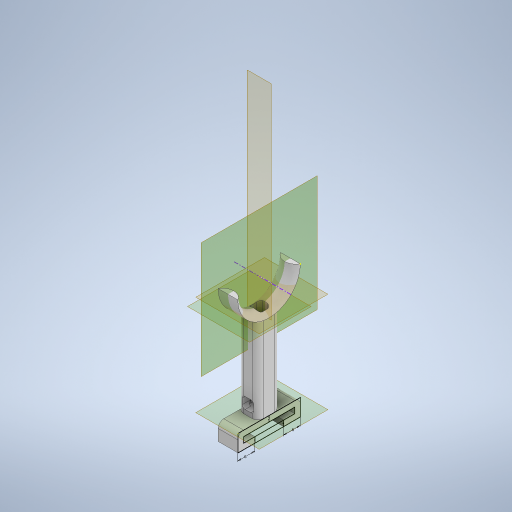
# Autodesk Inventor part: 막대1
Saved by Autodesk Inventor 2023 (Build 270158000, 158)
## iProperties
Created: 2023-04-26
Part Number: 막대1
Material: 일반
Document SubType Name: Modeling
Designer: rlatk
Density: 1 g/cm^3
Appearance: 기본값
Author: rlatk
Autodesk Inventor part; units mm, degrees
ref_plane "YZ Plane" through (0, 0, 0) normal (1, 0, 0) x (0, 1, 0)
ref_plane "XZ Plane" through (0, 0, 0) normal (0, 1, 0) x (-1, 0, 0)
sketch "스케치1" plane through (0, 0, 0) normal (0, 1, 0) x (-1, 0, 0)
  line L0 (0, 0) -> (3.5, 0)
  line L1 (0, 0) -> (-3.5, 0)
  arc A0 (3.5, 0) -> (-3.5, 0) centre (0, -1.9365) ccw
  line L2 (3.5, 0) -> (-3.5, 0)
  dimension "d1" = 3.5
  dimension "d2" = 4
  constraints: 6 end point, 2 point on circle, 1 centre point, 1 collinear, 1 horizontal
  measures "d1" distance of L0.start L0.end
  measures "d2" radius of A0
ref_plane "작업 평면4" through (0, 0, 11.1) normal (0, 0, 1) x (1, 0, 0)
sketch "스케치8" plane through (0, 0, 11.1) normal (0, 0, 1) x (1, 0, 0)
  point P0 (0, 0)
sketch "스케치9" plane through (0, 0, 11.1) normal (0, 0, 1) x (1, 0, 0)
  line L0 (11.2042, 0) -> (-9.3223, 0)
  point P0 (0, 0)
  constraints: 2 end point, 1 horizontal
revolve "회전2" add sketch "스케치1" angle 180 about axis through (11.2042, 0, 11.1) along (-1, 0, 0)
ref_plane "작업 평면5" through (-3.5, -11.1, 11.1) normal (0, -1, 0) x (1, 0, 0)
sketch "스케치10" plane through (-3.5, -11.1, 11.1) normal (0, -1, 0) x (1, 0, 0)
  line L0 (7, 11.1) -> (7, -11.1) projected
  line L1 (7, 0) -> (7, -4)
  line L2 (7, -4) -> (0, -4)
  line L3 (0, 11.1) -> (0, -11.1) projected
  line L4 (0, -4) -> (0, 0)
  line L5 (7, 0) -> (0, 0)
  line L6 (7, -11.1) -> (7, 11.1)
  line L7 (7, 4) -> (0, 4)
  line L8 (0, -11.1) -> (0, 11.1)
  point P0 (3.5, -11.1)
  point P1 (0, 4)
  dimension "d21" = 4
  constraints: 14 end point, 6 symmetric about line, 4 point on line, 2 midpoint, 2 perpendicular
  measures "d21" distance of L1.start L1.end
extrude "돌출4" add sketch "스케치10" along normal blind 30
ref_plane "작업 평면6" through (0, 0, 11.1) normal (-1, 0, 0) x (0, -1, 0)
sketch "스케치11" plane through (0, 0, 11.1) normal (-1, 0, 0) x (0, -1, 0)
  line L0 (11.1, -4) -> (11.1, 0) projected
  line L1 (11.1, -4) -> (10.3542, -4)
  arc A0 (0, -11.1) -> (11.1, 0) centre (0, 0) ccw projected
  line L2 (11.1, -4) -> (11.1, 0)
  arc A1 (10.3542, -4) -> (11.1, 0) centre (0, 0) ccw
  line L3 (11.1, 0) -> (9.0457, 0)
  line L4 (11.1, 4) -> (11.1, 0)
  line L5 (11.1, 4) -> (10.3542, 4)
  arc A2 (11.1, 0) -> (0, 11.1) centre (0, 0) ccw
  arc A3 (11.1, 0) -> (10.3542, 4) centre (0, 0) ccw
  constraints: 10 end point, 8 point on circle, 3 centre point, 3 symmetric about line, 2 horizontal, 1 collinear, 1 concentric, 1 tangent, 2 other
extrude "돌출5" add sketch "스케치11" along normal blind 3.5 and the other way blind 3.5
fillet "모깎기1" radius 2 4 edges at (-3.5, -25.7271, 15.1) (-3.5, -25.7271, 7.1) (3.5, -25.7271, 7.1) (3.5, -25.7271, 15.1)
ref_plane "작업 평면7" through (2.9142, -41.1, 14.5142) normal (0, -1, 0) x (1, 0, 0)
sketch "스케치12" plane through (2.9142, -41.1, 14.5142) normal (0, -1, 0) x (1, 0, 0)
  line L0 (0.5858, 7.6858) -> (0.5858, -1.4142) projected
  line L1 (-6.4142, -5.4142) -> (-6.4142, -14.5142) projected
  line L2 (0.5858, 7.6858) -> (-6.4142, 7.6858)
  line L3 (-6.4142, 7.6858) -> (-6.4142, -14.5142)
  line L4 (-6.4142, -14.5142) -> (0.5858, -14.5142)
  line L5 (0.5858, -14.5142) -> (0.5858, 7.6858)
  point P0 (-2.9142, -14.5142)
  point P1 (0.5858, -1.4142)
  constraints: 8 end point, 2 parallel, 1 horizontal, 1 perpendicular
extrude "돌출6" add sketch "스케치12" along normal blind 6
sketch "스케치13" plane through (3.5, 0, 11.1) normal (1, 0, 0) x (0, 0, -1)
  line L0 (-11.1, -41.1) -> (-11.1, -47.1) projected
  line L1 (11.1, -41.1) -> (11.1, -47.1) projected
  line L2 (-11.1, -41.1) -> (11.1, -41.1)
  line L3 (11.1, -41.1) -> (11.1, -47.1)
  line L4 (11.1, -47.1) -> (-11.1, -47.1)
  line L5 (-11.1, -47.1) -> (-11.1, -41.1)
  line L6 (11.1, -47.1) -> (-11.1, -47.1) projected
  line L7 (9.1, -43.1) -> (-9.1, -43.1)
  line L8 (-9.1, -43.1) -> (-9.1, -45.1)
  line L9 (-9.1, -45.1) -> (9.1, -45.1)
  line L10 (9.1, -45.1) -> (9.1, -43.1)
  line L11 (-5.1, -45.1) -> (-5.1, -47.1)
  line L12 (-11.1, -47.1) -> (11.1, -47.1) projected
  line L13 (5.1, -45.1) -> (5.1, -47.1)
  point P0 (11.1, 0)
  point P1 (-5.1, -46.1)
  point P2 (5.1, -46.1)
  point P3 (5.1, -47.1)
  point P4 (-5.1, -47.1)
  dimension "d38" = 2
  dimension "d39" = 6
  dimension "d40" = 6
  constraints: 20 end point, 5 parallel, 4 point on line, 3 perpendicular, 2 midpoint, 1 horizontal, 3 other
  measures "d38" distance between parallel lines of L2 L7
  measures "d39" distance from line of L0 point (-5.1, -46.1)
  measures "d40" distance from line of L1 point (5.1, -46.1)
extrude "돌출9" cut sketch "스케치13" against normal blind 10 contours L9 L8 L7 L10
extrude "돌출10" cut sketch "스케치13" against normal blind 10 contours L11 L9 L13 L4
fillet "모깎기2" radius 2 2 edges at (0, -41.1, 22.2) (0, -41.1, 0)
ref_plane "작업 평면8" through (0, 0, 11.1) normal (-1, 0, 0) x (0, -1, 0)
ref_plane "작업 평면10" through (0, -5.55, -1.9365) normal (0, 1, 0) x (1, 0, 0)
sketch "스케치14" plane through (0, -5.55, -1.9365) normal (0, 1, 0) x (1, 0, 0)
  point P0 (0, -1.9365)
sketch "스케치15" plane through (-3.5, -11.1, 11.1) normal (0, -1, 0) x (1, 0, 0)
  point P0 (3.5, -11.1)
sketch "스케치16" plane through (-3.5, -11.1, 11.1) normal (0, -1, 0) x (1, 0, 0)
  point P0 (3.5, -11.1)
sketch "스케치17" plane through (0, -5.55, -1.9365) normal (0, 1, 0) x (1, 0, 0)
  line L0 (-1, -15.0365) -> (1, -15.0365)
  line L1 (2, -14.0365) -> (2, -12.0365)
  line L2 (1, -11.0365) -> (-1, -11.0365)
  line L3 (-2, -12.0365) -> (-2, -14.0365)
  line L4 (15.3095, -13.0365) -> (-13.4276, -13.0365) projected
  line L5 (-3.5, -11.0365) -> (-3.5, -15.0365) projected
  arc A0 (-1, -11.0365) -> (-2, -12.0365) centre (-1, -12.0365) ccw
  arc A1 (-2, -14.0365) -> (-1, -15.0365) centre (-1, -14.0365) ccw
  arc A2 (1, -15.0365) -> (2, -14.0365) centre (1, -14.0365) ccw
  arc A3 (2, -12.0365) -> (1, -11.0365) centre (1, -12.0365) ccw
  point P0 (0, -1.9365)
  point P1 (-2, -15.0365)
  point P2 (2, -11.0365)
  point P3 (2, -15.0365)
  point P4 (-2, -11.0365)
  point P5 (2, -13.0365)
  point P6 (-2, -13.0365)
  point P7 (0, -11.0365)
  point P8 (0, -15.0365)
  dimension "d46" = 4
  dimension "d47" = 4
  dimension "d48" = 2
  dimension "d49" = 1.5
  dimension "d54" = 1
  constraints: 8 end point, 8 point on circle, 8 point on line, 8 tangent, 4 centre point, 4 midpoint, 3 equal radius, 2 parallel, 1 horizontal, 1 perpendicular
  measures "d46" distance of point (2, -13.036) point (-2, -13.036)
  measures "d47" distance from line of point (0, -11.036) L0
  measures "d48" distance from line of point (0, -15.036) L4
  measures "d49" distance between parallel lines of L3 L5
  measures "d54" radius of A0
extrude "돌출11" cut sketch "스케치17" against normal blind 34
sketch "스케치18" plane through (-1.5, -10.3542, 15.1) normal (0, 0, 1) x (1, 0, 0)
  line L0 (2.5, -29.1958) -> (0.5, -29.1958) projected
  line L1 (-0.5, 0.9931) -> (-0.5, -29.1958) projected
  line L2 (3.5, 0.9931) -> (3.5, -29.1958) projected
  line L3 (3.5, 0.9931) -> (3.5, -29.1958) projected
  line L4 (0.5, -25.1958) -> (2.5, -25.1958)
  line L5 (3.5, -26.1958) -> (3.5, -28.1958)
  line L6 (2.5, -29.1958) -> (0.5, -29.1958)
  line L7 (-0.5, -28.1958) -> (-0.5, -26.1958)
  arc A0 (0.5, -25.1958) -> (-0.5, -26.1958) centre (0.5, -26.1958) ccw
  arc A1 (-0.5, -28.1958) -> (0.5, -29.1958) centre (0.5, -28.1958) ccw
  arc A2 (2.5, -29.1958) -> (3.5, -28.1958) centre (2.5, -28.1958) ccw
  arc A3 (3.5, -26.1958) -> (2.5, -25.1958) centre (2.5, -26.1958) ccw
  point P0 (1.5, 10.3542)
  point P1 (-0.5, -25.1958)
  point P2 (-0.5, -26.1958)
  point P3 (-0.5, -28.1958)
  point P4 (3.5, -28.1958)
  dimension "d52" = 4
  dimension "d53" = 1
  constraints: 8 end point, 8 point on circle, 8 tangent, 5 point on line, 4 centre point, 3 equal radius, 2 parallel, 1 horizontal, 1 perpendicular
  measures "d52" distance between parallel lines of L0 L4
  measures "d53" radius of A0
extrude "돌출12" cut sketch "스케치18" against normal blind 3
